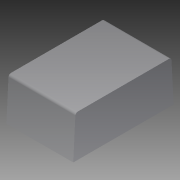
# Autodesk Inventor part: LED0603-Top
Saved by Autodesk Inventor 2015 SP1 (Build 190203100, 203)
## iProperties
Created: 2016-05-25
Part Number: LED0603-Top
Material: Generic
Document SubType Name: Modeling
Designer: danil
Density: 1 g/cm^3
Appearance: Default
Author: danil
Autodesk Inventor part; units mm, degrees
ref_plane "YZ Plane" through (0, 0, 0) normal (1, 0, 0) x (0, 1, 0)
ref_plane "XZ Plane" through (0, 0, 0) normal (0, 1, 0) x (-1, 0, 0)
ref_plane "XY Plane" through (0, 0, 0) normal (0, 0, 1) x (1, 0, 0)
sketch "Sketch1" plane through (0, 0, 0) normal (0, 0, 1) x (1, 0, 0)
  line L0 (0.4, -0.6) -> (-0.4, -0.6)
  line L1 (-0.4, -0.6) -> (-0.4, 0.6)
  line L2 (-0.4, 0.6) -> (0.4, 0.6)
  line L3 (0.4, 0.6) -> (0.4, -0.6)
  line L4 (0.4, -0.6) -> (-0.4, 0.6) construction
  line L5 (-0.4, -0.6) -> (0.4, 0.6) construction
  point P0 (0, 0)
  dimension "d0" = 0.8
  dimension "d1" = 1.2
  constraints: 12 end point, 2 midpoint, 2 parallel, 1 horizontal, 1 perpendicular
  measures "d0" distance of L1.end L2.end
  measures "d1" distance of L0.end L1.end
extrude "Extrusion1" add sketch "Sketch1" along normal blind 0.5
draft "FaceDraft1" angle -3 pull direction (0, 0, -1) faces at (0.1333, -0.6, 0.1667) fixed edges at (0, -0.6, 0)
draft "FaceDraft2" angle -3 pull direction (0, 0, -1) faces at (-0.1333, 0.6, 0.1667) fixed edges at (0, 0.6, 0)
fillet "Fillet1" radius 0.03 2 edges at (0, -0.5738, 0.5) (0, 0.5738, 0.5)
body "Solid1"
